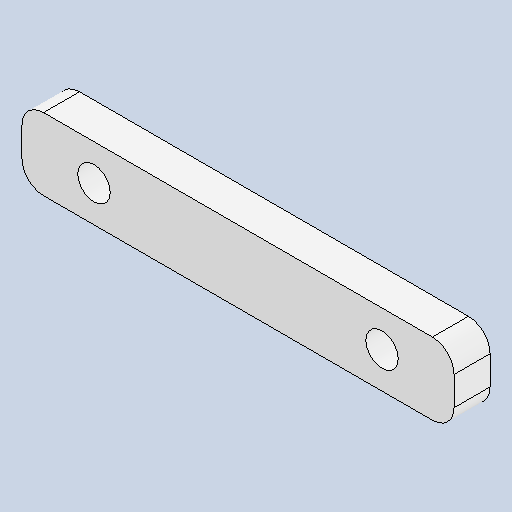
# Autodesk Inventor part: joint4_base_fixture
Saved by Autodesk Inventor 2025.3 (Build 293356030, 356C)
## iProperties
Created: 2025-11-09
Part Number: joint4_base_fixture
Material: PLA filament
Document SubType Name: Modeling
Designer: MSI
Mass: 3.36279 g
Surface Area: 19.3655 cm^2
Volume: 2.80233 cm^3
Density: 1.2 g/cm^3
Appearance: 일반
Author: MSI
Autodesk Inventor part; units mm, degrees
ref_plane "YZ Plane" through (0, 0, 0) normal (1, 0, 0) x (0, 1, 0)
ref_plane "XZ Plane" through (0, 0, 0) normal (0, 1, 0) x (-1, 0, 0)
ref_plane "XY Plane" through (0, 0, 0) normal (0, 0, 1) x (1, 0, 0)
sketch "스케치1" plane through (0, 0, 0) normal (0, 0, 1) x (1, 0, 0)
  line L0 (30, 5) -> (-30, 5)
  line L1 (-30, 5) -> (-30, -5)
  line L2 (-30, -5) -> (30, -5)
  line L3 (30, -5) -> (30, 5)
  line L4 (30, 5) -> (-30, -5) construction
  line L5 (-30, 5) -> (30, -5) construction
  point P0 (0, 0)
  dimension "d0" = 60
  dimension "d1" = 10
  constraints: 12 end point, 2 midpoint, 2 parallel, 1 horizontal, 1 perpendicular
  measures "d0" distance of L2.end L1.end
  measures "d1" distance of L1.end L0.end
extrude "돌출1" add sketch "스케치1" along normal mid plane 5
sketch "스케치2" plane through (0, 0, 2.5) normal (0, 0, 1) x (1, 0, 0)
  line L0 (-20, 0) -> (20, 0)
  point P0 (0, 0)
  point P1 (0, 0)
  dimension "d4" = 40
  constraints: 2 end point, 1 coincident, 1 horizontal, 1 midpoint
  measures "d4" distance of L0.start L0.end
hole "구멍1" at (20, 0, 2.5) at (-20, 0, 2.5) direction (0, 0, -1) diameter 4.5 end through all clearance for "Socket Head Cap Screw ISO 4762" size "M4" standard "ISO"
fillet "모깎기1" radius 3 4 edges at (30, 5, 0) (-30, 5, 0) (-30, -5, 0) (30, -5, 0)
